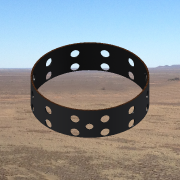
# Autodesk Inventor part: 2h1sout
Saved by Autodesk Inventor 2013 SP2 (Build 170200200, 200)
## iProperties
Company: HERA Project
Created: 2013-05-14
Part Number: 2h1sout
Material: Generic
Document SubType Name: Modeling
Designer: David DeBoer
Density: 1 g/cm^3
Description: Hub outer sonotube
Author: David DeBoer
Title: Hub outer sono
Autodesk Inventor part; units mm, degrees
ref_plane "YZ Plane" through (0, 0, 0) normal (1, 0, 0) x (0, 1, 0)
ref_plane "XZ Plane" through (0, 0, 0) normal (0, 1, 0) x (-1, 0, 0)
ref_plane "XY Plane" through (0, 0, 0) normal (0, 0, 1) x (1, 0, 0)
sketch "Sketch1" plane through (0, 0, 0) normal (0, 1, 0) x (-1, 0, 0)
  circle A0 centre (0, 0) radius 457.2
  circle A1 centre (0, 0) radius 444.5
  dimension "d0" = 914.4
  dimension "d2" = 12.7
  constraints: 2 centre point, 1 coincident
  measures "d0" diameter of A0
  measures "d2" radial gap between concentric circles of A1 A0
extrude "tube" add sketch "Sketch1" along normal blind 254
sketch "Sketch2" plane through (0, 0, 0) normal (0, -1, 0) x (1, 0, 0)
  circle A0 centre (0, 0) radius 444.5 projected
  circle A1 centre (0, 0) radius 457.2 projected
  point P0 (-457.2, 0)
  constraints: 1 horizontal alignment, 1 other
ref_plane "Work Plane1" through (-457.2, 0, 0) normal (-1, 0, 0) x (0, -1, 0)
sketch "Sketch3" plane through (-457.2, 0, 0) normal (-1, 0, 0) x (0, -1, 0)
  circle A0 centre (-162.56, 0) radius 12.7
  line L0 (0, -457.2) -> (0, 457.2) projected
  point P0 (0, 0)
  dimension "d5" = 25.4
  dimension "d7" = 162.56
  constraints: 1 centre point
  measures "d5" diameter of A0
  measures "d7" distance from line of A0.centre L0
hole "spar" at (-457.2, 162.56, 0) direction (1, 0, 0) diameter 73.025 end through all
pattern_circular "spar pattern" count 12 over 360 about axis through (0, 0, 0) along (0, 1, 0) of "spar"
sketch "Sketch4" plane through (0, 254, 0) normal (0, 1, 0) x (1, 0, 0)
  circle A0 centre (0, 0) radius 444.5 projected
  circle A1 centre (0, 0) radius 457.2 projected
  line L0 (-6.8782, 0) -> (527.6153, -106.3174) construction
  line L1 (-6.8782, 0) -> (538.0866, 0) construction
  point P0 (448.1513, -90.511)
  dimension "d18" = 11.25
  constraints: 4 end point, 1 equal length, 1 horizontal, 1 point on line, 2 other
  measures "d18" angle of L0 L1
ref_plane "Work Plane2" through (448.1513, 254, 90.511) normal (0.9807853, 0, 0.1950903) x (0, 1, 0)
sketch "Sketch7" plane through (-457.2, 0, 0) normal (-1, 0, 0) x (0, -1, 0)
  circle A0 centre (-38.1, 0) radius 30.1625
  point P0 (0, 0)
  dimension "d32" = 60.325
  dimension "d33" = 38.1
  constraints: 1 centre point
  measures "d32" diameter of A0
  measures "d33" distance of point (0, 0) A0.centre
hole "support" at (-457.2, 38.1, 0) direction (1, 0, 0) diameter 73.025 end through all
pattern_circular "support pattern" count 12 over 360 about axis through (0, 0, 0) along (0, 1, 0) of "support"
sketch "Sketch8" plane through (0, 254, 0) normal (0, 1, 0) x (1, 0, 0)
  circle A0 centre (0, 0) radius 444.5 projected
  circle A1 centre (0, 0) radius 457.2 projected
  point P0 (320.675, -325.8825)
  constraints: 2 other
ref_plane "Work Plane3" through (320.675, 254, 325.8825) normal (0.7013889, 0, 0.7127788) x (0, 1, 0)
sketch "Sketch9" plane through (320.675, 254, 325.8825) normal (0.7013889, 0, 0.7127788) x (0, 1, 0)
  circle A0 centre (-152.4, 0) radius 30.48
  point P0 (-254, 0)
  dimension "d44" = 60.96
  dimension "d45" = 101.6
  constraints: 1 centre point
  measures "d44" diameter of A0
  measures "d45" distance of point (-254, 0) A0.centre
extrude "conduit" cut sketch "Sketch9" against normal blind 25.4
body "Solid1"
